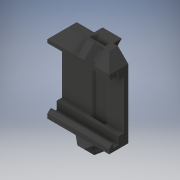
# Autodesk Inventor part: extruder_breakout_mount
Saved by Autodesk Inventor 2017 (Build 210142000, 142)
## iProperties
Created: 2017-06-16
Part Number: extruder_breakout_mount
Material: Generic
Document SubType Name: Modeling
Designer: yibre
Density: 1 g/cm^3
Appearance: Default
Author: yibre
Autodesk Inventor part; units mm, degrees
ref_plane "YZ Plane" through (0, 0, 0) normal (1, 0, 0) x (0, 1, 0)
ref_plane "XZ Plane" through (0, 0, 0) normal (0, 1, 0) x (-1, 0, 0)
ref_plane "XY Plane" through (0, 0, 0) normal (0, 0, 1) x (1, 0, 0)
ref_plane "Work Plane1" through (2, -31.725, -1.9) normal (1, 0, 0) x (0, 0, -1)
ref_plane "Work Plane3" through (11, -31.725, -5.9) normal (-1, 0, 0) x (0, 0, 1)
sketch "Sketch2" plane through (2, -31.725, -1.9) normal (1, 0, 0) x (0, 0, -1)
  line L0 (-6, 6.0325) -> (-7.5515, 6.0325) construction
  line L1 (-6, 29.4005) -> (-7.5515, 29.4005) construction
  line L2 (-7.5515, 29.4005) -> (-7.5515, 6.0325) construction
  line L3 (-6, 6.0325) -> (-6, 29.4005) construction
  line L4 (-7.8515, 5.3325) -> (-5.7, 5.3325)
  line L5 (-5.7, 5.3325) -> (-5.7, 30.1005)
  line L6 (-5.7, 30.1005) -> (-7.8515, 30.1005)
  line L7 (-7.8515, 30.1005) -> (-7.8515, 5.3325)
  line L8 (1.275, 0.1) -> (-1.9, 3.275)
  line L9 (-1.9, 31.725) -> (1.275, 34.9)
  line L10 (-1.9, 29) -> (-1.9, 31.725)
  line L11 (-1.9, 6) -> (-1.9, 29)
  line L12 (-1.9, 3.275) -> (-1.9, 6)
  line L13 (1.275, 34.9) -> (-9.3515, 34.9)
  line L14 (-9.3515, 34.9) -> (-9.3515, 0.1)
  line L15 (-9.3515, 0.1) -> (1.275, 0.1)
extrude "Extrusion2" add sketch "Sketch2" along normal up to surface (9 mm away)
sketch "Sketch3" plane through (2, -31.725, -1.9) normal (-1, 0, 0) x (0, 0, 1)
  line L0 (7.8515, 30.1005) -> (7.8515, 5.3325) projected
  line L1 (7.8515, 5.3325) -> (5.7, 5.3325) projected
  line L2 (5.7, 5.3325) -> (5.7, 30.1005) projected
  line L3 (5.7, 30.1005) -> (7.8515, 30.1005) projected
  line L4 (1.9, 31.725) -> (-1.275, 34.9) construction
  line L5 (1.9, 3.275) -> (1.9, 31.725) projected
  line L6 (-1.275, 0.1) -> (1.9, 3.275) construction
  line L7 (9.3515, 0.1) -> (-1.275, 0.1) projected
  line L8 (9.3515, 34.9) -> (9.3515, 0.1) projected
  line L9 (-1.275, 34.9) -> (9.3515, 34.9) projected
  line L10 (2, 2) -> (2, 33) projected
  line L11 (2, 33) -> (2, 34.9)
  line L12 (2, 2) -> (2, 0.1)
  point P0 (1.9, 31.725)
  constraints: 4 end point, 3 point on line, 1 vertical
extrude "Extrusion3" add sketch "Sketch3" along normal blind 10
sketch "Sketch4" plane through (11, -31.625, 7.4515) normal (1, 0, 0) x (0, 0, -1)
  line L0 (1.5, 5.2325) -> (3.6515, 5.2325) projected
  line L1 (3.6515, 5.2325) -> (3.6515, 30.0005) projected
  line L2 (3.6515, 30.0005) -> (1.5, 30.0005) projected
  line L3 (1.5, 30.0005) -> (1.5, 5.2325) projected
  line L4 (7.3515, 0) -> (0, 0) projected
  line L5 (0, 0) -> (0, 34.8) projected
  line L6 (0, 34.8) -> (7.3515, 34.8) projected
  line L7 (7.3515, 34.8) -> (7.3515, 0) projected
  point P0 (7.4515, 31.625)
extrude "Extrusion4" add sketch "Sketch4" along normal blind 5
sketch "Sketch5" plane through (-8, -31.625, 7.4515) normal (0, 0, 1) x (1, 0, 0)
  line L0 (0, 30.0005) -> (24, 30.0005) projected
  line L1 (0, 5.2325) -> (0, 30.0005) projected
  line L2 (0, 5.2325) -> (24, 5.2325) projected
  line L3 (24, 30.0005) -> (24, 5.2325) projected
  line L4 (0, 6.7325) -> (24, 6.7325)
  line L5 (24, 6.7325) -> (24, 28.5005)
  line L6 (24, 28.5005) -> (0, 28.5005)
  line L7 (0, 28.5005) -> (0, 6.7325)
  point P0 (8, 31.625)
  dimension "d18" = 1.5
  dimension "d19" = 1.5
  constraints: 8 end point, 2 parallel, 2 point on line, 1 horizontal, 1 perpendicular
  measures "d18" distance between parallel lines of L0 L6
  measures "d19" distance between parallel lines of L2 L4
extrude "Extrusion5" cut sketch "Sketch5" against normal up to next contours L6 L3 L4 L1
chamfer "Chamfer1" distance 1 angle 45 2 edges at (4, -3.1245, 7.4515) (4, -24.8925, 7.4515)
chamfer "Chamfer2" distance 4 angle 45 6 edges at (4, 3.175, 7.4515) (4, -31.625, 7.4515) (-8, -31.625, 3.7757) (-8, 3.175, 3.7757) (16, 3.175, 3.7757) (16, -31.625, 3.7757)
sketch "Sketch6" plane through (2, -31.625, -3.175) normal (0, -1, 0) x (1, 0, 0)
  line L0 (1.5, 5.675) -> (7.5, 5.675)
  line L1 (7.5, 5.675) -> (7.5, 4.175)
  line L2 (7.5, 4.175) -> (1.5, 4.175)
  line L3 (1.5, 4.175) -> (1.5, 5.675)
  line L4 (0, 0) -> (9, 0) projected
  line L5 (4.4809, 12.2555) -> (4.4809, 18.3515) projected
  line L6 (4.5, 4.175) -> (4.5, 0)
  point P0 (-2, 3.175)
  point P1 (0, 3.175)
  dimension "d28" = 6
  dimension "d29" = 1.5
  dimension "d53" = 1
  constraints: 10 end point, 2 midpoint, 2 parallel, 2 perpendicular, 1 horizontal
  measures "d28" distance of L1.end L2.end
  measures "d29" distance of L0.end L1.end
  measures "d53" distance from line of L2 point (0, 3.175)
extrude "Extrusion6" cut sketch "Sketch6" against normal through all
fillet "Fillet1" radius 2 2 edges at (6.5, -31.625, 1) (6.5, 3.175, 1)
sketch "Sketch7" plane through (16, -31.625, 7.4515) normal (1, 0, 0) x (0, 0, -1)
  line L0 (3.6515, 30.0005) -> (3.6515, 5.2325) projected
  line L1 (3.6515, 27.0005) -> (5.6515, 27.0005)
  line L2 (5.6515, 27.0005) -> (5.6515, 8.2325)
  line L3 (5.6515, 8.2325) -> (3.6515, 8.2325)
  line L4 (3.6515, 8.2325) -> (3.6515, 27.0005)
  line L5 (3.6515, 5.2325) -> (1.5, 5.2325) projected
  line L6 (1.5, 30.0005) -> (3.6515, 30.0005) projected
  point P0 (7.4515, 31.625)
  dimension "d34" = 3
  dimension "d35" = 3
  dimension "d36" = 2
  constraints: 8 end point, 2 parallel, 1 horizontal, 1 perpendicular, 1 point on line
  measures "d34" distance between parallel lines of L5 L3
  measures "d35" distance between parallel lines of L6 L1
  measures "d36" distance of L2.end L3.end
extrude "Extrusion7" cut sketch "Sketch7" against normal through all
move faces "Move1" translate (-0.8, 0, 0) faces at (11, -30.5667, -1.025)
move faces "Move2" translate (0.8, 0, 0) faces at (2, -30.5667, -1.025)
ref_plane "Work Plane4" through (6.5, -28.45, 0) normal (-1, 0, 0) x (0, 0, 1)
sketch "Sketch8" plane through (6.5, -28.45, 0) normal (-1, 0, 0) x (0, 0, 1)
  line L0 (7.4515, 27.625) -> (3.4515, 31.625) projected
  line L1 (6.6889, 28.3876) -> (4.214, 30.8624)
  line L2 (4.214, 30.8624) -> (5.0979, 31.7463)
  line L3 (5.0979, 31.7463) -> (7.5728, 29.2714)
  line L4 (7.5728, 29.2714) -> (6.6889, 28.3876)
  line L5 (7.4515, 27.625) -> (9.0425, 29.216)
  line L6 (9.0425, 29.216) -> (5.0425, 33.216)
  line L7 (5.0425, 33.216) -> (3.4515, 31.625)
  point P0 (0, 28.45)
  point P1 (5.4515, 29.625)
  dimension "d45" = 3.5
  dimension "d46" = 1.25
  dimension "d47" = 1
  constraints: 14 end point, 3 perpendicular, 2 midpoint, 2 parallel, 2 point on line
  measures "d45" distance of L1.start L1.end
  measures "d46" distance of L1.end L2.end
  measures "d47" distance between parallel lines of L6 L3
extrude "Extrusion8" add sketch "Sketch8" along normal mid plane 7 contours L0 L4 L3 L2 L7 L6 L5
ref_plane "Work Plane5" through (-8, -14.225, 20.8515) normal (0, 1, 0) x (-1, 0, 0)
mirror "Mirror1" about plane through (-8, -14.225, 20.8515) normal (0, 1, 0) of "Extrusion8"
chamfer "Chamfer3" distance 1 angle 45 6 edges at (3.5, -31.0392, 0.4142) (3.5, -14.225, 1) (3.5, 2.5892, 0.4142) (9.5, -31.0392, 0.4142) (9.5, -14.225, 1) (9.5, 2.5892, 0.4142)
chamfer "Chamfer4" distance 2.25 angle 45 4 edges at (3, -31.216, 7.0425) (10, -31.216, 7.0425) (3, 2.766, 7.0425) (10, 2.766, 7.0425)
body "Solid2"
